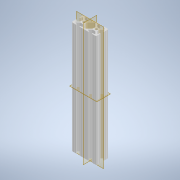
# Autodesk Inventor part: McMaster-Carr 47065T418 6
Saved by Autodesk Inventor 2022 (Build 260153000, 153)
## iProperties
Created: 2021-07-16
Part Number: McMaster-Carr 47065T418 6
Material: Generic
Document SubType Name: Modeling
Designer: negre
Density: 1 g/cm^3
Appearance: Default
Author: negre
Autodesk Inventor part; units mm, degrees
ref_plane "YZ Plane" through (0, 0, 0) normal (1, 0, 0) x (0, 1, 0)
ref_plane "XZ Plane" through (0, 0, 0) normal (0, 1, 0) x (-1, 0, 0)
sketch "Sketch1" plane through (0, 0, 0) normal (0, 1, 0) x (-1, 0, 0)
  circle A0 centre (14.8336, 12.7) radius 2.6035
  circle A1 centre (-10.5664, 12.7) radius 2.6035
  arc A2 (20.1507, 25.4) -> (21.1667, 25.4) centre (20.6587, 25.4) ccw
  line L0 (21.1667, 25.4) -> (24.384, 25.4)
  arc A3 (24.384, 25.4) -> (25.4, 25.3998) centre (24.892, 25.4) ccw
  arc A4 (27.5335, 23.2664) -> (25.4, 25.3998) centre (25.4254, 23.2918) ccw
  arc A5 (27.5335, 23.2664) -> (27.5336, 22.2504) centre (27.5336, 22.7584) ccw
  line L1 (27.5336, 22.2504) -> (27.5336, 19.0332)
  arc A6 (27.5336, 19.0332) -> (27.5336, 18.0171) centre (27.5336, 18.5251) ccw
  line L2 (27.5336, 18.0171) -> (27.5336, 16.9375)
  arc A7 (26.5346, 15.9385) -> (27.5336, 16.9375) centre (26.5346, 16.9375) ccw
  line L3 (26.5346, 15.9385) -> (26.3228, 15.9385)
  arc A8 (25.3238, 16.9375) -> (26.3228, 15.9385) centre (26.3228, 16.9375) ccw
  line L4 (25.3238, 16.9375) -> (25.3238, 19.3769)
  arc A9 (25.3238, 19.3769) -> (23.66, 20.0534) centre (24.3543, 19.3769) ccw
  line L5 (23.66, 20.0534) -> (20.243, 16.5465)
  arc A10 (20.243, 16.5465) -> (19.3421, 14.3308) centre (22.5171, 14.3308) ccw
  line L6 (19.3421, 14.3308) -> (19.3421, 11.0692)
  arc A11 (19.3421, 11.0692) -> (20.4318, 8.675) centre (22.5171, 11.0692) ccw
  line L7 (20.4318, 8.675) -> (23.7176, 5.8131)
  arc A12 (23.7176, 5.8131) -> (25.3238, 6.5441) centre (24.3543, 6.5441) ccw
  line L8 (25.3238, 6.5441) -> (25.3238, 8.4625)
  arc A13 (26.3228, 9.4615) -> (25.3238, 8.4625) centre (26.3228, 8.4625) ccw
  line L9 (26.3228, 9.4615) -> (26.5346, 9.4615)
  arc A14 (27.5336, 8.4625) -> (26.5346, 9.4615) centre (26.5346, 8.4625) ccw
  line L10 (27.5336, 8.4625) -> (27.5336, 7.3829)
  arc A15 (27.5336, 7.3829) -> (27.5336, 6.3669) centre (27.5336, 6.8749) ccw
  line L11 (27.5336, 6.3669) -> (27.5336, 3.1496)
  arc A16 (27.5336, 3.1496) -> (27.5335, 2.1336) centre (27.5336, 2.6416) ccw
  arc A17 (25.4, 0.0002) -> (27.5335, 2.1336) centre (25.4254, 2.1082) ccw
  arc A18 (25.4, 0.0002) -> (24.384, 0) centre (24.892, 0) ccw
  line L12 (24.384, 0) -> (21.1667, 0)
  arc A19 (21.1667, 0) -> (20.1507, 0) centre (20.6587, 0) ccw
  line L13 (20.1507, 0) -> (19.1211, 0)
  arc A20 (18.0721, 1.049) -> (19.1211, 0) centre (19.1211, 1.049) ccw
  line L14 (18.0721, 1.049) -> (18.0721, 1.1608)
  arc A21 (19.1211, 2.2098) -> (18.0721, 1.1608) centre (19.1211, 1.1608) ccw
  line L15 (19.1211, 2.2098) -> (21.25, 2.2098)
  arc A22 (21.25, 2.2098) -> (22.0019, 4.2178) centre (21.25, 3.3545) ccw
  line L16 (22.0019, 4.2178) -> (18.3215, 7.4234)
  arc A23 (18.3215, 7.4234) -> (16.2362, 8.2042) centre (16.2362, 5.0292) ccw
  line L17 (16.2362, 8.2042) -> (12.9746, 8.2042)
  arc A24 (12.9746, 8.2042) -> (10.7315, 7.2763) centre (12.9746, 5.0292) ccw
  line L18 (10.7315, 7.2763) -> (7.6143, 4.1647)
  arc A25 (7.6143, 4.1647) -> (8.423, 2.2098) centre (8.423, 3.3545) ccw
  line L19 (8.423, 2.2098) -> (10.5461, 2.2098)
  arc A26 (11.5952, 1.1608) -> (10.5461, 2.2098) centre (10.5461, 1.1608) ccw
  line L20 (11.5952, 1.1608) -> (11.5952, 1.049)
  arc A27 (10.5461, 0) -> (11.5952, 1.049) centre (10.5461, 1.049) ccw
  line L21 (10.5461, 0) -> (9.5165, 0)
  arc A28 (9.5165, 0) -> (8.5005, 0) centre (9.0085, 0) ccw
  line L22 (8.5005, 0) -> (5.2832, 0)
  arc A29 (5.2832, 0) -> (4.2672, 0) centre (4.7752, 0) ccw
  line L23 (4.2672, 0) -> (0, 0)
  arc A30 (0, 0) -> (-1.016, 0) centre (-0.508, 0) ccw
  line L24 (-1.016, 0) -> (-4.2333, 0)
  arc A31 (-4.2333, 0) -> (-5.2493, 0) centre (-4.7413, 0) ccw
  line L25 (-5.2493, 0) -> (-6.2789, 0)
  arc A32 (-7.3279, 1.049) -> (-6.2789, 0) centre (-6.2789, 1.049) ccw
  line L26 (-7.3279, 1.049) -> (-7.3279, 1.1608)
  arc A33 (-6.2789, 2.2098) -> (-7.3279, 1.1608) centre (-6.2789, 1.1608) ccw
  line L27 (-6.2789, 2.2098) -> (-4.15, 2.2098)
  arc A34 (-4.15, 2.2098) -> (-3.4323, 3.9449) centre (-4.15, 3.2258) ccw
  line L28 (-3.4323, 3.9449) -> (-6.7698, 7.2763)
  arc A35 (-6.7698, 7.2763) -> (-9.0128, 8.2042) centre (-9.0128, 5.0292) ccw
  line L29 (-9.0128, 8.2042) -> (-12.12, 8.2042)
  arc A36 (-12.12, 8.2042) -> (-14.363, 7.2763) centre (-12.12, 5.0292) ccw
  line L30 (-14.363, 7.2763) -> (-17.7005, 3.9449)
  arc A37 (-17.7005, 3.9449) -> (-16.9828, 2.2098) centre (-16.9828, 3.2258) ccw
  line L31 (-16.9828, 2.2098) -> (-14.8539, 2.2098)
  arc A38 (-13.8048, 1.1608) -> (-14.8539, 2.2098) centre (-14.8539, 1.1608) ccw
  line L32 (-13.8048, 1.1608) -> (-13.8048, 1.049)
  arc A39 (-14.8539, 0) -> (-13.8048, 1.049) centre (-14.8539, 1.049) ccw
  line L33 (-14.8539, 0) -> (-15.8835, 0)
  arc A40 (-15.8835, 0) -> (-16.8995, 0) centre (-16.3915, 0) ccw
  line L34 (-16.8995, 0) -> (-20.1168, 0)
  arc A41 (-20.1168, 0) -> (-21.1328, 0.0002) centre (-20.6248, 0) ccw
  arc A42 (-23.2662, 2.1336) -> (-21.1328, 0.0002) centre (-21.1582, 2.1082) ccw
  arc A43 (-23.2662, 2.1336) -> (-23.2664, 3.1496) centre (-23.2664, 2.6416) ccw
  line L35 (-23.2664, 3.1496) -> (-23.2664, 6.3669)
  arc A44 (-23.2664, 6.3669) -> (-23.2664, 7.3829) centre (-23.2664, 6.8749) ccw
  line L36 (-23.2664, 7.3829) -> (-23.2664, 8.4125)
  arc A45 (-22.2174, 9.4615) -> (-23.2664, 8.4125) centre (-22.2174, 8.4125) ccw
  line L37 (-22.2174, 9.4615) -> (-22.1056, 9.4615)
  arc A46 (-21.0566, 8.4125) -> (-22.1056, 9.4615) centre (-22.1056, 8.4125) ccw
  line L38 (-21.0566, 8.4125) -> (-21.0566, 6.202)
  arc A47 (-21.0566, 6.202) -> (-19.298, 5.4726) centre (-20.026, 6.202) ccw
  line L39 (-19.298, 5.4726) -> (-16.0069, 8.7577)
  arc A48 (-16.0069, 8.7577) -> (-15.0749, 11.0048) centre (-18.2499, 11.0048) ccw
  line L40 (-15.0749, 11.0048) -> (-15.0749, 14.2536)
  arc A49 (-15.0749, 14.2536) -> (-16.0143, 16.5082) centre (-18.2499, 14.2536) ccw
  line L41 (-16.0143, 16.5082) -> (-19.3004, 19.7665)
  arc A50 (-19.3004, 19.7665) -> (-21.0566, 19.0347) centre (-20.026, 19.0347) ccw
  line L42 (-21.0566, 19.0347) -> (-21.0566, 16.9875)
  arc A51 (-22.1056, 15.9385) -> (-21.0566, 16.9875) centre (-22.1056, 16.9875) ccw
  line L43 (-22.1056, 15.9385) -> (-22.2674, 15.9385)
  arc A52 (-23.2664, 16.9375) -> (-22.2674, 15.9385) centre (-22.2674, 16.9375) ccw
  line L44 (-23.2664, 16.9375) -> (-23.2664, 18.0171)
  arc A53 (-23.2664, 18.0171) -> (-23.2664, 19.0331) centre (-23.2664, 18.5251) ccw
  line L45 (-23.2664, 19.0331) -> (-23.2664, 22.2504)
  arc A54 (-23.2664, 22.2504) -> (-23.2662, 23.2664) centre (-23.2664, 22.7584) ccw
  arc A55 (-21.1328, 25.3998) -> (-23.2662, 23.2664) centre (-21.1582, 23.2918) ccw
  arc A56 (-21.1328, 25.3998) -> (-20.1168, 25.4) centre (-20.6248, 25.4) ccw
  line L46 (-20.1168, 25.4) -> (-16.8995, 25.4)
  arc A57 (-16.8995, 25.4) -> (-15.8835, 25.4) centre (-16.3915, 25.4) ccw
  line L47 (-15.8835, 25.4) -> (-14.8538, 25.4)
  arc A58 (-13.8049, 24.351) -> (-14.8538, 25.4) centre (-14.8538, 24.351) ccw
  line L48 (-13.8049, 24.351) -> (-13.8049, 24.2392)
  arc A59 (-14.8539, 23.1902) -> (-13.8049, 24.2392) centre (-14.8539, 24.2392) ccw
  line L49 (-14.8539, 23.1902) -> (-16.9828, 23.1902)
  arc A60 (-16.9828, 23.1902) -> (-17.7338, 21.3661) centre (-16.9828, 22.1235) ccw
  line L50 (-17.7338, 21.3661) -> (-14.4564, 18.1163)
  arc A61 (-14.4564, 18.1163) -> (-12.2209, 17.1958) centre (-12.2209, 20.3708) ccw
  line L51 (-12.2209, 17.1958) -> (-8.9119, 17.1958)
  arc A62 (-8.9119, 17.1958) -> (-6.6764, 18.1163) centre (-8.9119, 20.3708) ccw
  line L52 (-6.6764, 18.1163) -> (-3.399, 21.3661)
  arc A63 (-3.399, 21.3661) -> (-4.15, 23.1902) centre (-4.15, 22.1235) ccw
  line L53 (-4.15, 23.1902) -> (-6.2789, 23.1902)
  arc A64 (-7.3279, 24.2392) -> (-6.2789, 23.1902) centre (-6.2789, 24.2392) ccw
  line L54 (-7.3279, 24.2392) -> (-7.3279, 24.351)
  arc A65 (-6.2789, 25.4) -> (-7.3279, 24.351) centre (-6.2789, 24.351) ccw
  line L55 (-6.2789, 25.4) -> (-5.2493, 25.4)
  arc A66 (-5.2493, 25.4) -> (-4.2333, 25.4) centre (-4.7413, 25.4) ccw
  line L56 (-4.2333, 25.4) -> (-1.016, 25.4)
  arc A67 (-1.016, 25.4) -> (0, 25.4) centre (-0.508, 25.4) ccw
  line L57 (0, 25.4) -> (4.2672, 25.4)
  arc A68 (4.2672, 25.4) -> (5.2832, 25.4) centre (4.7752, 25.4) ccw
  line L58 (5.2832, 25.4) -> (8.5005, 25.4)
  arc A69 (8.5005, 25.4) -> (9.5165, 25.4) centre (9.0085, 25.4) ccw
  line L59 (9.5165, 25.4) -> (10.5462, 25.4)
  arc A70 (11.5951, 24.351) -> (10.5462, 25.4) centre (10.5462, 24.351) ccw
  line L60 (11.5951, 24.351) -> (11.5951, 24.2392)
  arc A71 (10.5461, 23.1902) -> (11.5951, 24.2392) centre (10.5461, 24.2392) ccw
  line L61 (10.5461, 23.1902) -> (8.423, 23.1902)
  arc A72 (8.423, 23.1902) -> (7.6978, 21.4627) centre (8.423, 22.1742) ccw
  line L62 (7.6978, 21.4627) -> (10.9506, 18.1472)
  arc A73 (10.9506, 18.1472) -> (13.2169, 17.1958) centre (13.2169, 20.3708) ccw
  line L63 (13.2169, 17.1958) -> (16.4785, 17.1958)
  arc A74 (16.4785, 17.1958) -> (18.7526, 18.1551) centre (16.4785, 20.3708) ccw
  line L64 (18.7526, 18.1551) -> (21.9777, 21.4652)
  arc A75 (21.9777, 21.4652) -> (21.25, 23.1902) centre (21.25, 22.1742) ccw
  line L65 (21.25, 23.1902) -> (19.1211, 23.1902)
  arc A76 (18.0721, 24.2392) -> (19.1211, 23.1902) centre (19.1211, 24.2392) ccw
  line L66 (18.0721, 24.2392) -> (18.0721, 24.351)
  arc A77 (19.1211, 25.4) -> (18.0721, 24.351) centre (19.1211, 24.351) ccw
  line L67 (19.1211, 25.4) -> (20.1507, 25.4)
  arc A78 (0.5879, 3.1272) -> (1.7004, 2.667) centre (1.7004, 4.2418) ccw
  line L68 (1.7004, 2.667) -> (2.5668, 2.667)
  arc A79 (2.5668, 2.667) -> (3.6794, 3.1272) centre (2.5668, 4.2418) ccw
  line L69 (3.6794, 3.1272) -> (9.3931, 8.8306)
  arc A80 (9.3931, 8.8306) -> (10.3251, 11.0777) centre (7.1501, 11.0777) ccw
  line L70 (10.3251, 11.0777) -> (10.3251, 14.3223)
  arc A81 (10.3251, 14.3223) -> (9.4165, 16.5459) centre (7.1501, 14.3223) ccw
  line L71 (9.4165, 16.5459) -> (3.8092, 22.2611)
  arc A82 (3.8092, 22.2611) -> (2.6851, 22.733) centre (2.6851, 21.1582) ccw
  line L72 (2.6851, 22.733) -> (1.7384, 22.733)
  arc A83 (1.7384, 22.733) -> (0.6296, 22.2765) centre (1.7384, 21.1582) ccw
  line L73 (0.6296, 22.2765) -> (-5.1184, 16.5768)
  arc A84 (-5.1184, 16.5768) -> (-6.0579, 14.3223) centre (-2.8829, 14.3223) ccw
  line L74 (-6.0579, 14.3223) -> (-6.0579, 11.0777)
  arc A85 (-6.0579, 11.0777) -> (-5.1259, 8.8306) centre (-2.8829, 11.0777) ccw
  line L75 (-5.1259, 8.8306) -> (0.5879, 3.1272)
  point P0 (2.1336, 12.7)
  constraints: 168 point on circle, 152 end point, 86 centre point
extrude "Extrusion1" add sketch "Sketch1" along normal blind 239.7252
ref_plane "Work Plane6" through (0, 228.6, 0) normal (0, 1, 0) x (1, 0, 0)
sketch "Sketch2" plane through (0, 228.6, 0) normal (0, 1, 0) x (1, 0, 0)
  line L0 (-29.773, 0.98) -> (25.3049, 0.98)
  line L1 (25.3049, 0.98) -> (25.3049, -26.4828)
  line L2 (25.3049, -26.4828) -> (-29.773, -26.4828)
  line L3 (-29.773, -26.4828) -> (-29.773, 0.98)
  point P0 (0, 0)
  constraints: 8 end point, 2 parallel, 1 horizontal, 1 perpendicular
extrude "Extrusion2" cut sketch "Sketch2" along normal through all
ref_plane "Work Plane7" through (0, 114.3, 0) normal (0, 1, 0) x (1, 0, 0)
ref_plane "Work Plane8" through (16.8995, 0, 12.7) normal (0, 0, 1) x (1, 0, 0)
ref_plane "Work Plane9" through (-2.1336, 0, 22.2504) normal (1, 0, 0) x (0, 0, -1)
body "Solid1"
